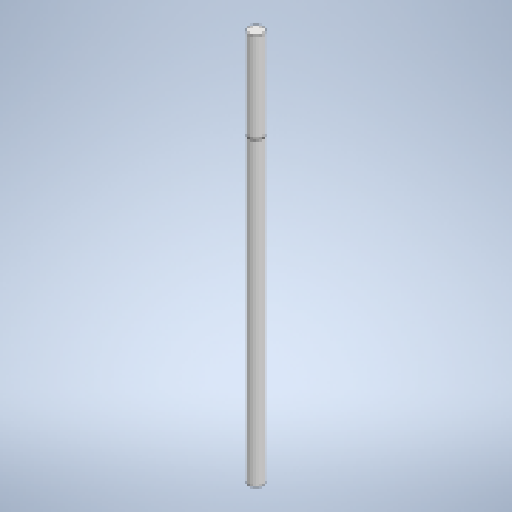
# Autodesk Inventor part: Вал
Saved by Autodesk Inventor 2025 (Build 290162010, 162A)
## iProperties
Created: 2024-04-09
Part Number: Вал
Material: Generic
Document SubType Name: Modeling
Designer: pokla
Density: 1 g/cm^3
Appearance: Default
Author: pokla
Autodesk Inventor part; units mm, degrees
ref_plane "YZ Plane" through (0, 0, 0) normal (1, 0, 0) x (0, 1, 0)
ref_plane "XZ Plane" through (0, 0, 0) normal (0, 1, 0) x (-1, 0, 0)
ref_plane "XY Plane" through (0, 0, 0) normal (0, 0, 1) x (1, 0, 0)
sketch "Sketch1" plane through (0, 0, 0) normal (1, 0, 0) x (0, 1, 0)
  line L0 (250, 0) -> (-250, 0)
  line L1 (-250, 0) -> (-250, -8.5)
  line L2 (-250, -8.5) -> (250, -8.5)
  line L3 (250, -8.5) -> (250, 0)
  line L4 (135, -8.5) -> (135, -7.5)
  line L5 (135, -7.5) -> (134, -7.5)
  line L6 (134, -7.5) -> (134, -8.5)
  line L7 (-212, -7.5) -> (-213, -7.5)
  line L8 (-213, -7.5) -> (-213, -8.5)
  line L9 (-213, -8.5) -> (-212, -8.5)
  line L10 (-212, -8.5) -> (-212, -7.5)
  point P0 (0, 0)
  point P1 (0, 0)
  point P2 (-212.5, -8.5)
  dimension "d0" = 500
  dimension "d1" = 8.5
  dimension "d2" = 1
  dimension "d3" = 1
  dimension "d4" = 115
  dimension "d6" = 1
  dimension "d7" = 1
  dimension "d8" = 462
  constraints: 22 end point, 4 parallel, 4 perpendicular, 2 horizontal, 2 midpoint, 2 point on line, 1 coincident, 1 horizontal alignment, 1 vertical
  measures "d0" distance of L2.end L1.end
  measures "d1" distance of L1.end L0.end
  measures "d2" distance of L4.start L4.end
  measures "d3" distance of L4.end L5.end
  measures "d4" distance between parallel lines of L3 L4
  measures "d6" distance of L9.end L7.start
  measures "d7" distance of L7.start L7.end
  measures "d8" distance between parallel lines of L3 L10
revolve "Revolution1" add sketch "Sketch1" angle 360 about axis through (0, 250, 0) along (0, -1, 0) contours L3 L2 L4 L5 L6 L10 L7 L8 L1 L0
equation "\"d6\" = d2"
equation "\"d7\" = d3"
body "Solid1"
